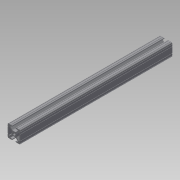
# Autodesk Inventor part: 1004
Saved by Autodesk Inventor 2013 (Build 170138000, 138)
## iProperties
Company: 80/20 Inc.
Created: 2014-04-23
Part Number: 1004
Material: Generic
Document SubType Name: Modeling
Density: 1 g/cm^3
Vendor: 80/20 Inc.
Engineer: Ross Bowman
Designer: Ross Bowman
Catalog Web Link: 8020.net
Material: 6105-T5 Aluminum
Author: Ross Bowman
Keywords: 80/20 , 8020 , T-Slot , Extrusion
Autodesk Inventor part; units mm, degrees
ref_plane "YZ Plane" through (0, 0, 0) normal (1, 0, 0) x (0, 1, 0)
ref_plane "XZ Plane" through (0, 0, 0) normal (0, 1, 0) x (-1, 0, 0)
ref_plane "XY Plane" through (0, 0, 0) normal (0, 0, 1) x (1, 0, 0)
sketch "Sketch1" plane through (0, 0, 0) normal (0, 0, 1) x (1, 0, 0)
  arc A0 (5.4405, 3.6206) -> (4.5085, 1.3735) centre (7.6835, 1.3735) ccw
  line L0 (9.0008, 7.1744) -> (5.4405, 3.6206)
  arc A1 (10.4902, 6.5567) -> (9.0008, 7.1744) centre (9.6174, 6.5567) ccw
  line L1 (10.4902, -6.5567) -> (10.4902, 6.5567)
  arc A2 (9.0008, -7.1744) -> (10.4902, -6.5567) centre (9.6174, -6.5567) ccw
  line L2 (5.4405, -3.6206) -> (9.0008, -7.1744)
  arc A3 (4.5085, -1.3735) -> (5.4405, -3.6206) centre (7.6835, -1.3735) ccw
  line L3 (4.5085, 1.3735) -> (4.5085, -1.3735)
  circle A4 centre (0, 0) radius 2.6035
  arc A5 (-9.0008, 7.1744) -> (-10.4902, 6.5567) centre (-9.6174, 6.5567) ccw
  line L4 (-5.4405, 3.6206) -> (-9.0008, 7.1744)
  arc A6 (-4.5085, 1.3735) -> (-5.4405, 3.6206) centre (-7.6835, 1.3735) ccw
  line L5 (-4.5085, -1.3735) -> (-4.5085, 1.3735)
  arc A7 (-5.4405, -3.6206) -> (-4.5085, -1.3735) centre (-7.6835, -1.3735) ccw
  line L6 (-9.0008, -7.1744) -> (-5.4405, -3.6206)
  arc A8 (-10.4902, -6.5567) -> (-9.0008, -7.1744) centre (-9.6174, -6.5567) ccw
  line L7 (-10.4902, 6.5567) -> (-10.4902, -6.5567)
  arc A9 (-7.3891, -8.6879) -> (-6.6435, -10.4902) centre (-6.6435, -9.4348) ccw
  line L8 (-7.3891, -8.6879) -> (-4.1189, -5.4237)
  arc A10 (-1.8759, -4.4958) -> (-4.1189, -5.4237) centre (-1.8759, -7.6708) ccw
  line L9 (-1.8759, -4.4958) -> (1.8759, -4.4958)
  arc A11 (4.1189, -5.4237) -> (1.8759, -4.4958) centre (1.8759, -7.6708) ccw
  line L10 (4.1189, -5.4237) -> (7.3891, -8.6879)
  arc A12 (6.6435, -10.4902) -> (7.3891, -8.6879) centre (6.6435, -9.4348) ccw
  line L11 (6.6435, -10.4902) -> (4.2875, -10.4902)
  arc A13 (4.2875, -10.4902) -> (3.2385, -11.5392) centre (4.2875, -11.5392) ccw
  line L12 (3.2385, -11.5392) -> (3.2385, -11.651)
  arc A14 (3.2385, -11.651) -> (4.2875, -12.7) centre (4.2875, -11.651) ccw
  line L13 (4.2875, -12.7) -> (5.3171, -12.7)
  arc A15 (6.3331, -12.7) -> (5.3171, -12.7) centre (5.8251, -12.7) ccw
  line L14 (6.3331, -12.7) -> (9.5504, -12.7)
  arc A16 (10.5664, -12.6998) -> (9.5504, -12.7) centre (10.0584, -12.7) ccw
  arc A17 (10.5664, -12.6998) -> (12.6998, -10.5664) centre (10.5918, -10.5918) ccw
  arc A18 (12.7, -9.5504) -> (12.6998, -10.5664) centre (12.7, -10.0584) ccw
  line L15 (12.7, -9.5504) -> (12.7, -6.3331)
  arc A19 (12.7, -5.3171) -> (12.7, -6.3331) centre (12.7, -5.8251) ccw
  line L16 (12.7, -5.3171) -> (12.7, 5.3171)
  arc A20 (12.7, 6.3331) -> (12.7, 5.3171) centre (12.7, 5.8251) ccw
  line L17 (12.7, 6.3331) -> (12.7, 9.5504)
  arc A21 (12.6998, 10.5664) -> (12.7, 9.5504) centre (12.7, 10.0584) ccw
  arc A22 (12.6998, 10.5664) -> (10.5664, 12.6998) centre (10.5918, 10.5918) ccw
  arc A23 (9.5504, 12.7) -> (10.5664, 12.6998) centre (10.0584, 12.7) ccw
  line L18 (9.5504, 12.7) -> (6.3331, 12.7)
  arc A24 (5.3171, 12.7) -> (6.3331, 12.7) centre (5.8251, 12.7) ccw
  line L19 (5.3171, 12.7) -> (4.2875, 12.7)
  arc A25 (4.2875, 12.7) -> (3.2385, 11.651) centre (4.2875, 11.651) ccw
  line L20 (3.2385, 11.651) -> (3.2385, 11.5392)
  arc A26 (3.2385, 11.5392) -> (4.2875, 10.4902) centre (4.2875, 11.5392) ccw
  line L21 (4.2875, 10.4902) -> (6.6858, 10.4902)
  arc A27 (7.419, 8.7178) -> (6.6858, 10.4902) centre (6.6858, 9.4523) ccw
  line L22 (7.419, 8.7178) -> (4.1189, 5.4237)
  arc A28 (1.8759, 4.4958) -> (4.1189, 5.4237) centre (1.8759, 7.6708) ccw
  line L23 (1.8759, 4.4958) -> (-1.8759, 4.4958)
  arc A29 (-4.1189, 5.4237) -> (-1.8759, 4.4958) centre (-1.8759, 7.6708) ccw
  line L24 (-4.1189, 5.4237) -> (-7.419, 8.7178)
  arc A30 (-6.6858, 10.4902) -> (-7.419, 8.7178) centre (-6.6858, 9.4523) ccw
  line L25 (-6.6858, 10.4902) -> (-4.2875, 10.4902)
  arc A31 (-4.2875, 10.4902) -> (-3.2385, 11.5392) centre (-4.2875, 11.5392) ccw
  line L26 (-3.2385, 11.5392) -> (-3.2385, 11.651)
  arc A32 (-3.2385, 11.651) -> (-4.2875, 12.7) centre (-4.2875, 11.651) ccw
  line L27 (-4.2875, 12.7) -> (-5.3171, 12.7)
  arc A33 (-6.3331, 12.7) -> (-5.3171, 12.7) centre (-5.8251, 12.7) ccw
  line L28 (-6.3331, 12.7) -> (-9.5504, 12.7)
  arc A34 (-10.5664, 12.6998) -> (-9.5504, 12.7) centre (-10.0584, 12.7) ccw
  arc A35 (-10.5664, 12.6998) -> (-12.6998, 10.5664) centre (-10.5918, 10.5918) ccw
  arc A36 (-12.7, 9.5504) -> (-12.6998, 10.5664) centre (-12.7, 10.0584) ccw
  line L29 (-12.7, 9.5504) -> (-12.7, 6.3331)
  arc A37 (-12.7, 5.3171) -> (-12.7, 6.3331) centre (-12.7, 5.8251) ccw
  line L30 (-12.7, 5.3171) -> (-12.7, -5.3171)
  arc A38 (-12.7, -6.3331) -> (-12.7, -5.3171) centre (-12.7, -5.8251) ccw
  line L31 (-12.7, -6.3331) -> (-12.7, -9.5504)
  arc A39 (-12.6998, -10.5664) -> (-12.7, -9.5504) centre (-12.7, -10.0584) ccw
  arc A40 (-12.6998, -10.5664) -> (-10.5664, -12.6998) centre (-10.5918, -10.5918) ccw
  arc A41 (-9.5504, -12.7) -> (-10.5664, -12.6998) centre (-10.0584, -12.7) ccw
  line L32 (-9.5504, -12.7) -> (-6.3331, -12.7)
  arc A42 (-5.3171, -12.7) -> (-6.3331, -12.7) centre (-5.8251, -12.7) ccw
  line L33 (-5.3171, -12.7) -> (-4.2875, -12.7)
  arc A43 (-4.2875, -12.7) -> (-3.2385, -11.651) centre (-4.2875, -11.651) ccw
  line L34 (-3.2385, -11.651) -> (-3.2385, -11.5392)
  arc A44 (-3.2385, -11.5392) -> (-4.2875, -10.4902) centre (-4.2875, -11.5392) ccw
  line L35 (-4.2875, -10.4902) -> (-6.6435, -10.4902)
  constraints: 88 point on circle, 72 end point, 45 centre point
extrude "Extrusion1" add sketch "Sketch1" against normal blind 304.8
body "Solid1"
